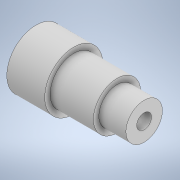
# Autodesk Inventor part: Peça5-Rubia
Saved by Autodesk Inventor 2021 (Build 250183000, 183)
## iProperties
Created: 2021-03-18
Part Number: Peça5-Rubia
Material: Genérico
Document SubType Name: Modeling
Designer: rubia
Density: 1 g/cm^3
Appearance: Padrão
Author: rubia
Autodesk Inventor part; units mm, degrees
ref_plane "YZ Plane" through (0, 0, 0) normal (1, 0, 0) x (0, 1, 0)
ref_plane "XZ Plane" through (0, 0, 0) normal (0, 1, 0) x (-1, 0, 0)
ref_plane "XY Plane" through (0, 0, 0) normal (0, 0, 1) x (1, 0, 0)
sketch "Esboço1" plane through (0, 0, 0) normal (0, 0, 1) x (1, 0, 0)
  line L0 (0, 0) -> (100, 0)
  line L1 (100, 0) -> (100, 10)
  line L2 (100, 10) -> (75, 10)
  line L3 (75, 10) -> (75, 15)
  line L4 (75, 15) -> (35, 15)
  line L5 (35, 15) -> (35, 20)
  line L6 (35, 20) -> (0, 20)
  line L7 (0, 0) -> (0, 20)
  line L8 (0, 0) -> (0, -6.8435) construction
  line L9 (0, -6.8435) -> (100, -6.8435) construction
  dimension "d1" = 100
  dimension "d2" = 10
  dimension "d3" = 25
  dimension "d4" = 5
  dimension "d5" = 40
  dimension "d6" = 5
  constraints: 20 end point, 5 perpendicular, 3 vertical, 2 horizontal
  measures "d1" distance of L0.start L0.end
  measures "d2" distance of L0.end L1.end
  measures "d3" distance of L1.end L2.end
  measures "d4" distance of L2.end L3.end
  measures "d5" distance of L3.end L4.end
  measures "d6" distance of L4.end L5.end
revolve "Revolução1" add sketch "Esboço1" angle 360 about axis through (0, -6.8435, 0) along (1, 0, 0)
sketch "Esboço3" plane through (0, -6.8435, 0) normal (-1, 0, 0) x (0, 0, 1)
  circle A0 centre (0, 0) radius 6.8435 projected
  circle A1 centre (0, 0) radius 10
  point P0 (0, 6.8435)
  dimension "d8" = 20
  constraints: 1 centre point, 1 coincident, 1 vertical alignment
  measures "d8" diameter of A1
extrude "Extrusão1" cut sketch "Esboço3" against normal blind 10 contours A0 | A1
